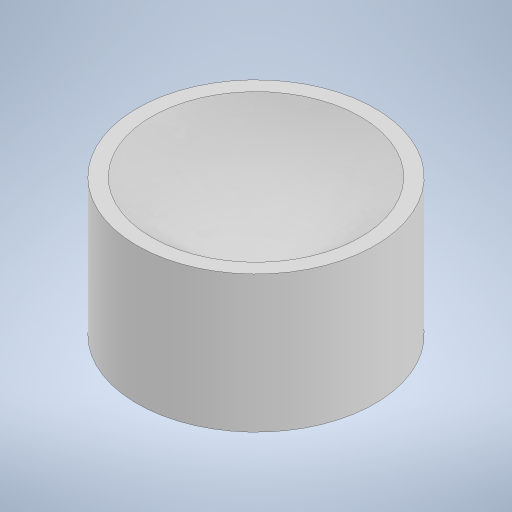
# Autodesk Inventor part: Goma tacómetro_v2.1
Saved by Autodesk Inventor 2023 (Build 270158000, 158)
## iProperties
Created: 2023-07-25
Part Number: Goma tacómetro_v2.1
Material: Generic
Document SubType Name: Modeling
Designer: checo
Density: 1 g/cm^3
Appearance: Default
Author: checo
Autodesk Inventor part; units mm, degrees
ref_plane "YZ Plane" through (0, 0, 0) normal (1, 0, 0) x (0, 1, 0)
ref_plane "XZ Plane" through (0, 0, 0) normal (0, 1, 0) x (-1, 0, 0)
ref_plane "XY Plane" through (0, 0, 0) normal (0, 0, 1) x (1, 0, 0)
sketch "Sketch1" plane through (0, 0, 0) normal (0, 1, 0) x (-1, 0, 0)
  circle A0 centre (0, 0) radius 7.5
  circle A1 centre (0, 0) radius 4.75
  circle A2 centre (0, 0) radius 14.25
  circle A3 centre (0, 0) radius 16.5
  line L0 (-4.6435, -1) -> (-7.433, -1)
  line L1 (0, 0) -> (-16.5, 0) construction
  line L2 (-4.6435, 1) -> (-7.433, 1)
  line L3 (1, -4.6435) -> (1, -7.433)
  line L4 (-1, -4.6435) -> (-1, -7.433)
  line L5 (4.6435, 1) -> (7.433, 1)
  line L6 (4.6435, -1) -> (7.433, -1)
  line L7 (-1, 4.6435) -> (-1, 7.433)
  line L8 (1, 4.6435) -> (1, 7.433)
  dimension "d1" = 15
  dimension "d2" = 9.5
  dimension "d3" = 33
  dimension "d0" = 28.5
  dimension "d7" = 1
  dimension "d10" = 360
  constraints: 18 end point, 4 coincident, 2 horizontal, 2 symmetric about line, 1 centre point, 1 horizontal alignment, 33 other
  measures "d0" diameter of A2
  measures "d7" distance from line of point (0, 0) L0
extrude "Extrusion1" add sketch "Sketch1" against normal blind 6 contours A3
extrude "Extrusion2" add sketch "Sketch1" along normal blind 5 contours L5 A1 L8 A0 | A0 L3 A1 L6 | L7 A1 L2 A0 | A0 L0 A1 L4 | A2 | A3
sketch "Sketch3" plane through (0, 0, 0) normal (1, 0, 0) x (0, 1, 0)
  line L0 (5, 16.5) -> (13, 16.5)
  line L1 (13, 16.5) -> (13, 14.5)
  line L2 (5, 0) -> (6.278, 0)
  arc A0 (13, 14.5) -> (6.278, 0) centre (25.278, 0) ccw
  line L3 (6.278, 0) -> (5, 0) construction
  line L4 (5, -16.5) -> (5, 16.5) projected
  line L5 (5, 16.5) -> (5, 0) construction
  line L6 (5, 0) -> (12, 0) construction
  point P0 (0, 0)
  dimension "d20" = 2
  dimension "d21" = 8
  dimension "d22" = 19
  constraints: 12 end point, 2 collinear, 2 horizontal, 2 point on circle, 2 point on line, 1 centre point, 1 midpoint, 1 perpendicular
  measures "d20" distance of L0.end L1.end
  measures "d21" distance of L0.start L0.end
  measures "d22" radius of A0
revolve "Revolution1" add sketch "Sketch3" angle 360 about axis through (0, 5, 0) along (0, 1, 0)
body "Solid1"
